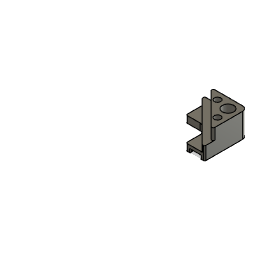
Corner Support (Autodesk Fusion 360 design; units mm, degrees)
Autodesk Fusion 360 part; units mm, degrees
sketch "Sketch1" plane through (0, 0, 0) normal (0, 1, 0) x (1, 0, 0)
  line L0 (125, 125) -> (-125, 125) construction
  line L1 (-125, 125) -> (-125, -125) construction
  line L2 (-125, -125) -> (125, -125) construction
  line L3 (125, -125) -> (125, 125) construction
  line L4 (125, 125) -> (-125, -125) construction
  line L5 (-125, 125) -> (125, -125) construction
  line L6 (75, 112.1152) -> (-75, 112.1152) construction
  line L7 (-75, 112.1152) -> (-75, 91.9152) construction
  line L8 (-75, 91.9152) -> (75, 91.9152) construction
  line L9 (75, 91.9152) -> (75, 112.1152) construction
  line L10 (75, 112.1152) -> (-75, 91.9152) construction
  line L11 (-75, 112.1152) -> (75, 91.9152) construction
  line L12 (137, 137) -> (92, 137)
  line L13 (92, 137) -> (137, 92)
  line L14 (137, 92) -> (137, 137)
  line L15 (125, 125) -> (137, 137) construction
  line L16 (128, 128) -> (109, 128) construction
  line L17 (109, 128) -> (128, 109) construction
  line L18 (128, 109) -> (128, 128) construction
  line L19 (92, 137) -> (84, 137)
  line L20 (84, 137) -> (84, 114)
  line L21 (84, 114) -> (104, 114)
  line L22 (104, 114) -> (114, 104)
  line L23 (114, 104) -> (114, 84)
  line L24 (114, 84) -> (137, 84)
  line L25 (137, 84) -> (137, 92)
  line L26 (84, 138) -> (-84, 138)
  line L27 (-84, 138) -> (-84, 113)
  line L28 (-84, 113) -> (84, 113)
  line L29 (84, 113) -> (84, 138)
  line L30 (84, 138) -> (-84, 113) construction
  line L31 (-84, 138) -> (84, 113) construction
  point P0 (0, 102.0152)
  point P1 (0, 125.5)
  dimension "d4" = 250
  dimension "d5" = 250
  dimension "d6" = 150
  dimension "d7" = 20.2
  dimension "d8" = 12
  dimension "d9" = 12
  dimension "d10" = 45
  dimension "d11" = 16
  dimension "d12" = 3
  dimension "d13" = 8
  dimension "d14" = 23
  dimension "d15" = 20
  dimension "d16" = 25
  dimension "d17" = 1
  constraint horizontal L0
  constraint perpendicular L0 L1
  constraint parallel L0 L2
  constraint parallel L1 L3
  constraint coincident L4 origin
  constraint coincident L5 origin
  constraint horizontal L6
  constraint perpendicular L6 L7
  constraint parallel L6 L8
  constraint parallel L7 L9
  constraint coincident L10 P0
  constraint coincident L11 P0
  constraint vertical origin P0
  constraint perpendicular L3 L12
  constraint perpendicular L4 L13
  constraint perpendicular L12 L14
  constraint parallel L4 L15
  constraint coincident L15 L16.start
  constraint parallel L12 L16
  constraint perpendicular L15 L17
  constraint perpendicular L16 L18
  constraint parallel L0 L19
  constraint perpendicular L0 L20
  constraint perpendicular L20 L21
  constraint parallel L13 L22
  constraint perpendicular L21 L23
  constraint perpendicular L23 L24
  constraint perpendicular L24 L25
  constraint equal L19 L25
  constraint equal L20 L24
  constraint horizontal L26
  constraint perpendicular L26 L27
  constraint parallel L26 L28
  constraint parallel L27 L29
  constraint coincident L30 P1
  constraint coincident L31 P1
  constraint coincident L20 L26.start
  constraint vertical origin P1
  measures "d4" distance of L1.end L2.end
  measures "d5" distance of L0.start L2.end
  measures "d6" distance of L6.start L6.end
  measures "d7" distance of L6 L8
  measures "d8" distance of L0 L12
  measures "d9" distance of L3 L14
  measures "d10" distance of L12.start L13.end
  measures "d11" horizontal distance of L0.start L16.end
  measures "d12" distance of L0 L16
  measures "d13" distance of L12.end L19.end
  measures "d14" distance of L19.end L20.end
  measures "d15" distance of L22.end L23.end
  measures "d16" distance of L26 L28
  measures "d17" distance of L19 L26
ref_plane "WorkPlane1" through (0, 8, 0) normal (0, 1, 0) x (0, 0, 1)
extrude "Extrude2" add sketch "Sketch1" along normal blind 16.25 contours L13 L19 L20 L21 L22 L23 L24 L25 L29
extrude "Extrude3" add sketch "Sketch1" along normal blind 30 contours L12 L13 L14
sketch "Sketch2" plane through (0, 30, 0) normal (0, 1, 0) x (-1, 0, 0)
  line L0 (-137, -92) -> (-137, -137)
  line L1 (-137, -137) -> (-92, -137)
  line L2 (-92, -137) -> (-137, -92)
  point P0 (-109, -128)
  point P1 (-128, -109)
sketch "Sketch4" plane through (0, 30, 0) normal (0, 1, 0) x (-1, 0, 0)
  line L0 (-137, -92) -> (-137, -137)
  line L1 (-137, -137) -> (-92, -137)
  line L2 (-92, -137) -> (-137, -92)
  point P0 (-128, -128)
  point P1 (-125, -125)
hole "Hole2" at (125, 30, -125) direction (0, -1, 0) diameter 6.2 end through all counterbore diameter 14 counterbore depth 26
sketch "Sketch5" plane through (0, 30, 0) normal (0, 1, 0) x (-1, 0, 0)
  line L0 (-137, -92) -> (-137, -137)
  line L1 (-137, -137) -> (-92, -137)
  line L2 (-92, -137) -> (-137, -92)
  circle A0 centre (-125, -125) radius 7
  point P0 (-109, -128)
  point P1 (-128, -109)
hole "Hole3" at (109, 30, -128) at (128, 30, -109) direction (0, -1, 0) diameter 7.9 depth 13.7 tip angle 180
sketch "Sketch9" plane through (0, 0, 0) normal (0, -1, 0) x (1, 0, 0)
  line L0 (84, -137) -> (137, -137)
  line L1 (137, -137) -> (137, -84)
  line L2 (137, -84) -> (114, -84)
  line L3 (114, -84) -> (114, -104)
  line L4 (114, -104) -> (104, -114)
  line L5 (104, -114) -> (84, -114)
  line L6 (84, -114) -> (84, -137)
  line L7 (84, -119.5) -> (90, -118)
  line L8 (90, -118) -> (90, -133)
  line L9 (90, -133) -> (84, -131.5)
  line L10 (90, -125.5) -> (84, -125.5) construction
  line L11 (84, -119.5) -> (90, -133) construction
  line L12 (84, -131.5) -> (90, -118) construction
  circle A0 centre (125, -125) radius 3.1
  dimension "d51" = 12
  dimension "d52" = 15
  dimension "d53" = 6
  constraint coincident L6 L7.start
  constraint parallel L6 L8
  constraint coincident L6 L9.end
  constraint midpoint L8 L10.start
  constraint midpoint L6 L10.end
  constraint horizontal L10
  constraint equal L11 L12
  measures "d51" distance of L7.start L9.end
  measures "d52" distance of L7.end L8.end
  measures "d53" distance of L7.start L8
extrude "Extrude7" cut sketch "Sketch9" against normal blind 4.4 contours L6 L7 L8 L9
fillet "Fillet1" radius 1 2 edges at (84, 2.2, -119.5) (84, 2.2, -131.5)
fillet "Fillet1" radius 1 2 edges at (90, 2.2, -118) (90, 2.2, -133)
ref_plane "WorkPlane2" through (137, 15, -137) normal (0.707107, 0, 0.707107) x (0, 1, 0)
mirror "Mirror2" about plane through (137, 15, -137) normal (0.707107, 0, 0.707107) of "Extrude7", "Fillet1"
sketch "Sketch10" plane through (0, 16.25, 0) normal (0, 1, 0) x (-1, 0, 0)
  line L0 (-92, -137) -> (-84, -137)
  line L1 (-84, -137) -> (-84, -114)
  line L2 (-84, -114) -> (-104, -114)
  line L3 (-104, -114) -> (-114, -104)
  line L4 (-114, -104) -> (-114, -84)
  line L5 (-114, -84) -> (-137, -84)
  line L6 (-137, -84) -> (-137, -92)
  line L7 (-137, -92) -> (-92, -137)
  line L8 (-84, -134) -> (-134, -84)
  constraint coincident L1 L8.start
  constraint parallel L3 L8
  constraint coincident L2.end L8
extrude "Extrude8" cut sketch "Sketch10" against normal blind 8 contours L1 L2 L8 | L4 L5 L8
fillet "Fillet2" radius 6 1 edges at (137, 15, -137)
fillet "Fillet3" radius 2 2 edges at (92, 23.125, -137) (137, 23.125, -92)
fillet "Fillet4" radius 6 2 edges at (104, 4.125, -114) (114, 4.125, -104)
fillet "Fillet5" radius 1.5 6 edges at (84, 8.125, -137) (84, 12.25, -134) (84, 4.125, -114) (114, 4.125, -84) (134, 12.25, -84) (137, 8.125, -84)
equation "sensor_ref = 8 mm"
